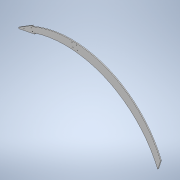
# Autodesk Inventor part: spoke3
Saved by Autodesk Inventor 2020.3 (Build 243373000, 373)
## iProperties
Created: 2020-11-01
Part Number: spoke3
Material: Generic
Document SubType Name: Modeling
Designer: Martijn
Density: 1 g/cm^3
Appearance: Default
Mass: 104.035 g
Surface Area: 584.811 cm^2
Volume: 104.035 cm^3
Author: Martijn
Autodesk Inventor part; units mm, degrees
ref_plane "YZ Plane" through (0, 0, 0) normal (1, 0, 0) x (0, 1, 0)
ref_plane "XZ Plane" through (0, 0, 0) normal (0, 1, 0) x (-1, 0, 0)
ref_plane "XY Plane" through (0, 0, 0) normal (0, 0, 1) x (1, 0, 0)
sketch "Sketch1" plane through (0, 0, 0) normal (0, 0, 1) x (1, 0, 0)
  arc A0 (670.9948, -199.4141) -> (0, 0) centre (254.9219, -370.8299) ccw
  arc A1 (657.7848, -239.4141) -> (30, 0) centre (229.3296, -420.1103) ccw
  arc A2 (657.7848, -239.4141) -> (670.9948, -199.4141) centre (0, 0) ccw
  line L0 (0, 0) -> (30, 0)
  line L1 (657.7848, -239.4141) -> (0, 0)
  line L2 (-143.7228, 0) -> (862.3369, 0) projected
  point P0 (0, 0)
  dimension "d1" = 30
  dimension "d2" = 40
  dimension "d4" = 20
  dimension "d5" = 465
  dimension "d6" = 450
  dimension "d22" = 700
  constraints: 6 point on circle, 4 end point, 3 centre point, 1 coincident, 1 horizontal
  measures "d1" distance of L0.start L0.end
  measures "d2" vertical distance of L1.start A0.start
  measures "d4" angle of L1 L2
  measures "d5" radius of A1
  measures "d6" radius of A0
  measures "d22" radius of A2
extrude "Extrusion1" add sketch "Sketch1" along normal blind 4 contours A2 A1 L2 A0 | L2 A1 L0 A0
sketch "Sketch2" plane through (0, 0, 4) normal (0, 0, 1) x (1, 0, 0)
  arc A0 (670.9948, -199.4141) -> (0, 0) centre (254.9219, -370.8299) ccw projected
  arc A1 (87.1309, 22.5434) -> (74.166, 50.9844) centre (0, 0) ccw
  line L0 (74.166, 50.9844) -> (0, 0)
  line L1 (0, 0) -> (87.1309, 22.5434)
  line L2 (0, 0) -> (30, 0) projected
  point P0 (78.8927, 43.3122)
  point P1 (0, 0)
  point P2 (0, 0)
  dimension "d9" = 90
  dimension "d16" = 20
  constraints: 4 end point, 2 point on circle, 1 centre point, 1 coincident, 1 tangent
  measures "d9" distance of L2.start L1.end
  measures "d16" angle of L1 L0
extrude "Extrusion2" add sketch "Sketch2" against normal blind 4
sketch "Sketch4" plane through (0, 0, 4) normal (0, 0, 1) x (1, 0, 0)
  line L0 (86.0304, 22.2587) -> (87.1309, 22.5434) projected
  line L1 (74.166, 50.9844) -> (0, 0) projected
  line L2 (87.1309, 22.5434) -> (0, 0)
  line L3 (0, 0) -> (30, 0)
  arc A0 (86.0304, 22.2587) -> (30, 0) centre (229.3296, -420.1103) ccw projected
  line L4 (30, 0) -> (86.0304, 22.2587)
  point P0 (86.0304, 22.2587)
  constraints: 6 end point, 1 horizontal
extrude "Extrusion4" cut sketch "Sketch4" against normal blind 10 contours A0 L3 L2
sketch "Sketch6" plane through (0, 0, 4) normal (0, 0, 1) x (1, 0, 0)
  circle A0 centre (71.4659, 35.9531) radius 1.5
  circle A1 centre (76.6234, 22.9969) radius 1.5
  circle A2 centre (37.1637, 14.7938) radius 1.5
  line L0 (0, 0) -> (87.1309, 22.5434) projected
  line L1 (37.1637, 14.7938) -> (0, 0)
  line L2 (0, 0) -> (71.4659, 35.9531)
  line L3 (74.166, 50.9844) -> (0, 0) projected
  line L4 (76.6234, 22.9969) -> (0, 0)
  circle A3 centre (264.574, 53.8573) radius 1.5
  circle A4 centre (260.1726, 72.1818) radius 1.5
  line L5 (261.3927, 67.6302) -> (0, 0)
  line L6 (264.574, 53.8573) -> (0, 0)
  circle A5 centre (281.2279, 70.1567) radius 1.5
  circle A6 centre (285.6292, 51.8321) radius 1.5
  line L7 (264.574, 53.8573) -> (260.1726, 72.1818)
  line L8 (281.2279, 70.1567) -> (260.1726, 72.1818)
  line L9 (281.2279, 70.1567) -> (285.6292, 51.8321)
  line L10 (285.6292, 51.8321) -> (264.574, 53.8573)
  line L11 (260.1726, 72.1818) -> (0, 0)
  dimension "d23" = 7.2
  dimension "d24" = 2.2
  dimension "d25" = 7.8
  dimension "d26" = 80
  dimension "d27" = 80
  dimension "d28" = 40
  dimension "d29" = 3
  dimension "d30" = 3
  dimension "d31" = 3
  dimension "d34" = 3
  dimension "d35" = 3
  dimension "d36" = 3
  dimension "d38" = 270
  dimension "d39" = 270
  dimension "d40" = 109
  dimension "d41" = 3
  dimension "d42" = 3
  dimension "d43" = 20
  dimension "d47" = 1
  dimension "d48" = 270
  constraints: 20 end point, 7 centre point, 2 parallel, 1 collinear
  measures "d23" angle of L1 L0
  measures "d24" angle of L0 L4
  measures "d25" angle of L2 L3
  measures "d26" distance of L0.start L2.end
  measures "d27" distance of L4.start L0.start
  measures "d28" distance of L1.start L0.start
  measures "d29" diameter of A0
  measures "d30" diameter of A1
  measures "d31" diameter of A2
  measures "d34" diameter of A4
  measures "d35" diameter of A3
  measures "d36" angle of L5 L6
  measures "d38" distance of L5.start L0.start
  measures "d39" distance of L6.start L0.start
  measures "d40" angle of L7 L10
  measures "d41" diameter of A6
  measures "d42" diameter of A5
  measures "d43" distance between parallel lines of L7 L9
  measures "d47" angle of L5 L11
  measures "d48" distance of L7.end L0.start
extrude "Extrusion6" cut sketch "Sketch6" against normal blind 10 from surface at 0 contours A0 | A1 | A2 | L6 L10 A3 | A3 L7 L6 | L11 L7 A4 | A4 L8 L11 | A3 L10 L7 | L7 L8 A4 | L10 L9 A6 | A6 L9 L10 | L8 L9 A5 | A5 L9 L8
sketch "Sketch7" plane through (0, 0, 4) normal (0, 0, 1) x (1, 0, 0)
  line L0 (87.1309, 22.5434) -> (0, 0) projected
  circle A0 centre (0, 0) radius 15
  dimension "d44" = 30
  constraints: 1 centre point, 1 coincident
  measures "d44" diameter of A0
extrude "Extrusion7" cut sketch "Sketch7" against normal blind 10
sketch "Sketch8" plane through (0, 0, 4) normal (0, 0, 1) x (1, 0, 0)
  arc A0 (78.8927, 43.3122) -> (74.166, 50.9844) centre (0, 0) ccw projected
  line L0 (74.166, 50.9844) -> (0, 0)
  line L1 (12.361, 8.4974) -> (74.166, 50.9844) projected
  line L2 (0, 0) -> (82.5313, 50.9844)
  line L3 (82.5313, 50.9844) -> (74.166, 50.9844)
  point P0 (76.568, 47.3005)
  dimension "d49" = 2.8
  constraints: 6 end point, 1 collinear, 1 horizontal
  measures "d49" angle of L2 L0
extrude "Extrusion8" cut sketch "Sketch8" against normal blind 10 contours L2 L0 A0
sketch "Sketch9" plane through (0, 0, 4) normal (0, 0, 1) x (1, 0, 0)
  line L0 (14.5218, 3.7572) -> (87.1309, 22.5434)
  line L1 (87.1309, 22.5434) -> (14.5218, 3.7572) projected
  arc A0 (14.688, 3.0434) -> (14.5218, 3.7572) centre (0, 0) ccw
  line L2 (14.688, 3.0434) -> (88.1281, 18.2602)
  arc A1 (88.1281, 18.2602) -> (87.1309, 22.5434) centre (0, 0) ccw
  line L3 (14.688, 3.0434) -> (0, 0)
  line L4 (0, 0) -> (14.5218, 3.7572)
  arc A2 (78.8927, 43.3122) -> (76.568, 47.3005) centre (0, 0) ccw projected
  dimension "d52" = 2.8
  constraints: 9 end point, 4 point on circle, 2 centre point, 2 coincident, 2 concentric, 1 collinear, 1 point on line
  measures "d52" angle of L0 L2
extrude "Extrusion9" add sketch "Sketch9" against normal blind 4 contours L0 A1 L2 A0
body "Solid1"
